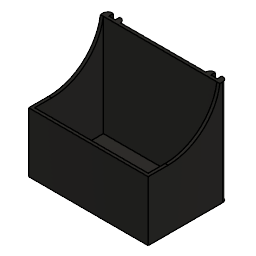
Caja_Receptora_Simple (Autodesk Fusion 360 design; units mm, degrees)
Autodesk Fusion 360 part; units mm, degrees
sketch "Boceto1" plane through (0, 0, 0) normal (0, 1, 0) x (1, 0, 0)
  line L0 (0, 0) -> (80, 0)
  line L1 (80, 0) -> (80, -50)
  line L2 (80, -50) -> (0, -50)
  line L3 (0, -50) -> (0, 0)
  line L4 (78, -48) -> (2, -48)
  line L5 (2, -48) -> (2, -2)
  line L6 (2, -2) -> (78, -2)
  line L7 (78, -2) -> (78, -48)
  dimension "d1" = 80
  dimension "d2" = 50
  dimension "d3" = 2
  constraint horizontal L0
  constraint vertical L1
  constraint horizontal L2
  constraint vertical L3
  constraint coincident L0.start L3.end
  measures "d1" distance of L0.start L0.end
  measures "d2" distance of L0.start L2.end
extrude "Extruir1" add sketch "Boceto1" along normal blind 40
extrude "Extruir2" add sketch "Boceto1" along normal blind 2 contours L4 L5 L6 L7
sketch "Boceto2" plane through (0, 40, 0) normal (0, 1, 0) x (-1, 0, 0)
  line L0 (-2, 2) -> (-78, 2)
  line L1 (-78, 2) -> (-78, 48)
  line L2 (-78, 48) -> (-2, 48)
  line L3 (-2, 48) -> (-2, 2)
  line L4 (0, 50) -> (-80, 50)
  line L5 (-80, 50) -> (-80, 0)
  line L6 (-80, 0) -> (0, 0)
  line L7 (0, 0) -> (0, 50)
  line L8 (-2, 2) -> (0, 2)
  line L9 (-78, 2) -> (-80, 2)
  constraint coincident L0.start L3.end
  constraint coincident L7 L8.end
  constraint perpendicular L7 L8
  constraint coincident L0.end L1.start
  constraint coincident L5 L9.end
  constraint perpendicular L5 L9
extrude "Extruir3" add sketch "Boceto2" along normal blind 30 contours L0 L5 L6 L7 L8 L9
fillet "Empalme1" radius 35 2 edges at (1, 40, 2) (79, 40, 2)
sketch "Boceto3" plane through (0, 0, 0) normal (0, 0, -1) x (-1, 0, 0)
  line L0 (-80, 0) -> (0, 0)
  line L1 (0, 0) -> (0, 70)
  line L2 (0, 70) -> (-80, 70)
  line L3 (-80, 70) -> (-80, 0)
  line L4 (-40, 70) -> (-72, 70)
  line L5 (-40, 70) -> (-8, 70)
  line L6 (-72, 70) -> (-76.3, 70)
  line L7 (-76.3, 70) -> (-76.3, 0)
  line L8 (-76.3, 0) -> (-72, 0)
  line L9 (-72, 0) -> (-72, 70)
  line L10 (-8, 70) -> (-3.7, 70)
  line L11 (-3.7, 70) -> (-3.7, 0)
  line L12 (-3.7, 0) -> (-8, 0)
  line L13 (-8, 0) -> (-8, 70)
  line L14 (-72, 70) -> (-68.5, 70)
  line L15 (-68.5, 70) -> (-68.5, 0)
  line L16 (-68.5, 0) -> (-72, 0)
  line L17 (-72, 0) -> (-72, 70)
  line L18 (-8, 70) -> (-11.5, 70)
  line L19 (-11.5, 70) -> (-11.5, 0)
  line L20 (-11.5, 0) -> (-8, 0)
  line L21 (-8, 0) -> (-8, 70)
  dimension "d12" = 32
  dimension "d13" = 32
  dimension "d14" = 4.3
  dimension "d15" = 4.3
  dimension "d16" = 3.5
  dimension "d17" = 3.5
  constraint midpoint L2 L4.start
  constraint parallel L2 L4
  constraint parallel L2 L5
  constraint horizontal L6
  constraint vertical L7
  constraint horizontal L8
  constraint vertical L9
  constraint horizontal L10
  constraint vertical L11
  constraint horizontal L12
  constraint vertical L13
  constraint horizontal L14
  constraint vertical L15
  constraint horizontal L16
  constraint vertical L17
  constraint horizontal L18
  constraint vertical L19
  constraint horizontal L20
  constraint vertical L21
  measures "d12" distance of L4.start L4.end
  measures "d13" distance of L4.start L5.end
  measures "d14" distance of L4.end L6.end
  measures "d15" distance of L5.end L10.end
  measures "d16" distance of L4.end L14.end
  measures "d17" distance of L5.end L18.end
extrude "Extruir4" add sketch "Boceto3" along normal blind 3 contours L0 L2 L3 L7 | L0 L2 L4 L9 L14 L15 L16 L17 | L0 L2 L5 L13 L18 L19 L20 L21 | L0 L1 L2 L11
fillet "Empalme2" radius 3 4 edges at (80, 35, -3) (68.5, 35, -3) (11.5, 35, -3) (0, 35, -3)
named bodies: "Caja Receptora"
